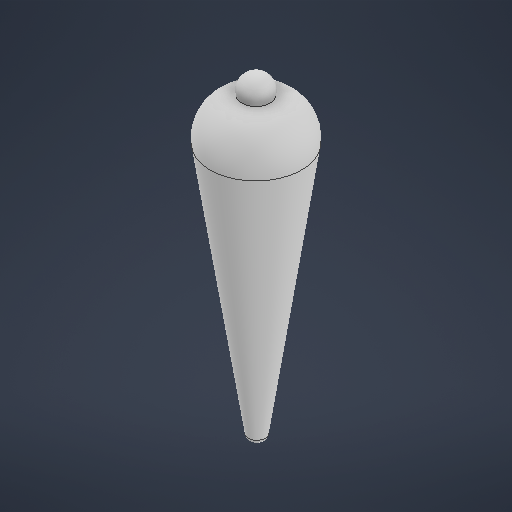
# Autodesk Inventor part: Leg
Saved by Autodesk Inventor 2025.2 (Build 292293000, 293)
## iProperties
Created: 2025-03-31
Part Number: Leg
Material: Generic
Document SubType Name: Modeling
Designer: mylap
Density: 1 g/cm^3
Appearance: Default
Author: mylap
## iProperties of the stored document Leg_3DPrint.ipt
Created: 2025-03-31
Part Number: Leg_3DPrint
Material: Generic
Document SubType Name: Modeling
Designer: mylap
Density: 1 g/cm^3
Appearance: Default
Author: mylap
Autodesk Inventor part; units mm, degrees
ref_plane "YZ Plane" through (0, 0, 0) normal (1, 0, 0) x (0, 1, 0)
ref_plane "XZ Plane" through (0, 0, 0) normal (0, 1, 0) x (-1, 0, 0)
ref_plane "XY Plane" through (0, 0, 0) normal (0, 0, 1) x (1, 0, 0)
sketch "Sketch1" plane through (0, 0, 0) normal (0, 0, 1) x (1, 0, 0)
  line L0 (3.9915, -2.7998) -> (48.4415, -2.7998) construction
  line L1 (48.4415, -2.7998) -> (48.4415, -85.3498) construction
  line L2 (48.4415, -85.3498) -> (3.9915, -85.3498) construction
  line L3 (3.9915, -85.3498) -> (3.9915, -2.7998) construction
  line L4 (16.0219, -56.9317) -> (24.9697, -56.9317)
  line L5 (24.9697, -56.9317) -> (21.3072, -82.0788)
  line L6 (20.8045, -82.5136) -> (20.3601, -82.5136)
  line L7 (19.8579, -82.0821) -> (16.0219, -56.9317)
  arc A0 (19.8579, -82.0821) -> (20.3601, -82.5136) centre (20.3601, -82.0056) ccw
  arc A1 (20.8045, -82.5136) -> (21.3072, -82.0788) centre (20.8045, -82.0056) ccw
  circle A2 centre (20.4958, -56.5507) radius 1.27
  line L8 (20.4958, -55.2807) -> (20.5823, -82.5136)
  point P0 (0, 0)
  point P1 (20.4958, -56.9317)
  point P2 (21.7073, -56.9317)
  point P3 (20.5038, -57.8206)
  dimension "d2" = 2.54
  dimension "d1" = 0.508
  dimension "d3" = 0.381
  dimension "d5" = 0
  constraints: 10 end point, 4 point on circle, 4 tangent, 2 centre point, 2 midpoint, 1 equal radius, 1 horizontal, 1 parallel, 5 other
  measures "d1" radius of A0
  measures "d3" distance of point (20.496, -56.551) point (20.496, -56.932)
  measures "d5" horizontal distance of point (20.496, -56.932) point (20.496, -56.551)
revolve "Revolution1" add sketch "Sketch1" angle 360 about axis through (20.4958, -55.2807, 0) along (0.0031771, -0.999995, 0) contours A2 L4 L5 A1 L6 L8
sketch "Sketch2" plane through (0, 0, 0) normal (0, 0, 1) x (1, 0, 0)
  circle A0 centre (20.4998, -56.5649) radius 1.27
  line L0 (16.0324, -56.9601) -> (24.9697, -56.9317) projected
  line L1 (19.2298, -56.5649) -> (21.7698, -56.5649)
  point P0 (0, 0)
  dimension "d8" = 2.54
  dimension "d9" = 0.381
  constraints: 2 end point, 2 point on circle, 1 centre point, 1 horizontal
  measures "d8" diameter of A0
  measures "d9" distance from line of L0 A0.centre
revolve "Revolution3" add sketch "Sketch2" angle 360 about axis through (19.2298, -56.5649, 0) along (1, 0, 0) contours L1 A0
fillet "Fillet1" radius 3.175 1 edges at (16.0324, -56.9601, 0)
body "Solid1"
